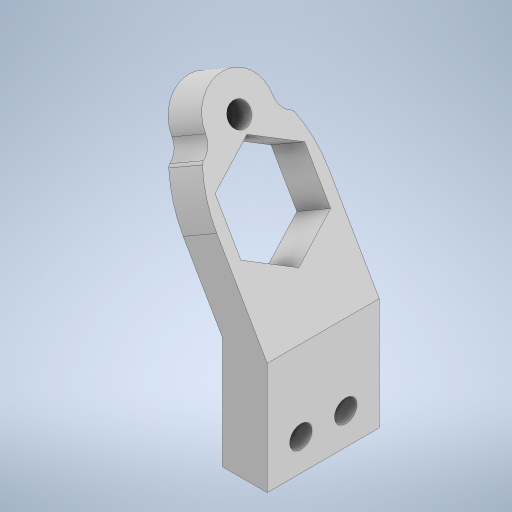
# Autodesk Inventor part: 6 - Part  5
Saved by Autodesk Inventor 2024 (Build 280153000, 153)
## iProperties
Created: 2024-04-21
Part Number: 6 - Part  5
Material: Generic
Document SubType Name: Modeling
Designer: Ricsi
Density: 1 g/cm^3
Appearance: Default
Author: Ricsi
Autodesk Inventor part; units mm, degrees
ref_plane "YZ Plane" through (0, 0, 0) normal (1, 0, 0) x (0, 1, 0)
ref_plane "XZ Plane" through (0, 0, 0) normal (0, 1, 0) x (-1, 0, 0)
ref_plane "XY Plane" through (0, 0, 0) normal (0, 0, 1) x (1, 0, 0)
sketch "Sketch1" plane through (0, 0, 0) normal (1, 0, 0) x (0, 1, 0)
  line L0 (28.0764, 57.8828) -> (-21.9236, 57.8828)
  line L1 (-21.9236, 57.8828) -> (-21.9236, 7.8828)
  line L2 (-21.9236, 7.8828) -> (28.0764, 7.8828)
  line L3 (28.0764, 7.8828) -> (28.0764, 57.8828)
  circle A0 centre (-7.7792, 22.8828) radius 5
  circle A1 centre (-7.7792, 42.8828) radius 5
  point P0 (0, 0)
  dimension "d0" = 50
  dimension "d1" = 50
  dimension "d3" = 10
  dimension "d5" = 10
  constraints: 8 end point, 2 centre point, 2 parallel, 1 horizontal, 1 perpendicular
  measures "d0" distance of L2.end L1.end
  measures "d1" distance of L1.end L0.end
  measures "d3" diameter of A0
  measures "d5" diameter of A1
extrude "Extrusion1" add sketch "Sketch1" along normal blind 20
sketch "Sketch2" plane through (0, -21.9236, 57.8828) normal (0, 0, 1) x (1, 0, 0)
  line L0 (20, 0) -> (20, 50) projected
  line L1 (20, 50) -> (-25, 127.9423)
  line L2 (20, 50) -> (110, 50) construction
  line L3 (0, 50) -> (-45, 127.9423)
  line L4 (0, 50) -> (90, 50) construction
  line L5 (-45, 127.9423) -> (-25, 127.9423)
  line L6 (0, 50) -> (20, 50)
  point P0 (0, 21.9236)
  dimension "d8" = 90
  dimension "d9" = 120
  dimension "d10" = 90
  dimension "d11" = 120
  constraints: 12 end point, 2 equal length, 2 horizontal, 1 collinear
  measures "d8" distance of L0.end L1.end
  measures "d9" angle of L2 L1
  measures "d10" distance of L3.start L3.end
  measures "d11" angle of L4 L3
extrude "Extrusion2" add sketch "Sketch2" against normal blind 50
sketch "Sketch3" plane through (20, 28.0764, 57.8828) normal (0.866, 0.5, 0) x (0, 0, -1)
  line L0 (0, 0) -> (0, -43.3013) projected
  line L1 (0, 0) -> (0, 90) projected
  arc A0 (40, 75) -> (10, 75) centre (25, 75) ccw
  line L2 (0, 0) -> (0, 45)
  line L3 (50, 0) -> (0, 0) projected
  line L4 (0, 0) -> (50, 0)
  line L5 (50, 0) -> (50, 45)
  arc A1 (5.4018, 67.7593) -> (10, 75) centre (2, 75) ccw
  line L6 (10, 75) -> (2, 75) construction
  line L7 (4.7362, 67.4825) -> (2, 75) construction
  arc A2 (40, 75) -> (44.5982, 67.7593) centre (48, 75) ccw
  line L8 (40, 75) -> (48, 75) construction
  line L9 (45.2638, 67.4825) -> (48, 75) construction
  arc A3 (4.4105, 66.7289) -> (0, 45) centre (55.73, 45) ccw
  arc A4 (50, 45) -> (45.5895, 66.7289) centre (-5.73, 45) ccw
  arc A5 (5.4018, 67.7593) -> (4.4105, 66.7289) centre (6.2523, 65.9491) ccw
  arc A6 (45.5895, 66.7289) -> (44.5982, 67.7593) centre (43.7477, 65.9491) ccw
  line L10 (25, 90) -> (0, 90)
  line L11 (0, 90) -> (0, 45)
  line L12 (50, 90) -> (50, 0) projected
  line L13 (50, 90) -> (50, 45)
  line L14 (25, 90) -> (50, 90)
  point P0 (57.8828, -14.3149)
  dimension "d18" = 45
  dimension "d19" = 45
  dimension "d20" = 8
  dimension "d21" = 70
  dimension "d22" = 8
  dimension "d23" = 70
  dimension "d24" = 2
  dimension "d25" = 2
  constraints: 22 end point, 20 point on circle, 9 tangent, 7 centre point, 2 collinear, 2 midpoint, 2 perpendicular
  measures "d18" distance of L0.start L2.end
  measures "d19" distance of L3.start L5.end
  measures "d20" radius of A1
  measures "d21" angle of L7 L6
  measures "d22" radius of A2
  measures "d23" angle of L8 L9
  measures "d24" radius of A5
  measures "d25" radius of A6
extrude "Extrusion3" cut sketch "Sketch3" against normal blind 50 contours L1 L10 A0 A1 A5 A3 | A4 A6 A2 A0 L14 L12
sketch "Sketch4" plane through (-40, 97.3585, 32.8828) normal (0.5, -0.866, 0) x (0.866, 0.5, 0)
  line L0 (17.3205, 25) -> (17.3205, 0) projected
  line L1 (17.3205, 0) -> (17.3205, -25) projected
  line L2 (17.3205, 25) -> (17.3205, -25)
  line L3 (17.3205, -25) -> (-0.3461, -25)
  line L4 (-0.3461, -25) -> (-0.3461, 25)
  line L5 (17.3205, 25) -> (0, 25) projected
  line L6 (-0.3461, 25) -> (17.3205, 25)
  point P0 (-14.0382, -32.8828)
  point P1 (0, 25)
  constraints: 8 end point, 3 perpendicular, 1 collinear
extrude "Extrusion4" cut sketch "Sketch4" against normal blind 50
sketch "Sketch5" plane through (20, 28.0764, 57.8828) normal (0.866, 0.5, 0) x (0, 0, -1)
  line L0 (50, 0) -> (0, 0) projected
  circle A0 centre (25, 75) radius 5
  point P0 (57.8828, -14.3149)
  dimension "d32" = 10
  constraints: 1 centre point
  measures "d32" diameter of A0
extrude "Extrusion5" cut sketch "Sketch5" against normal blind 50
sketch "Sketch6" plane through (20, 28.0764, 57.8828) normal (0.866, 0.5, 0) x (0, 0, -1)
  line L0 (0, 0) -> (0, 45) projected
  line L1 (50, 0) -> (0, 0) projected
  line L2 (25, 68.094) -> (45, 56.547)
  line L3 (45, 56.547) -> (45, 33.453)
  line L4 (45, 33.453) -> (25, 21.906)
  line L5 (25, 21.906) -> (5, 33.453)
  line L6 (5, 33.453) -> (5, 56.547)
  line L7 (5, 56.547) -> (25, 68.094)
  point P0 (57.8828, -14.3149)
  point P1 (25, 45)
  point P2 (45, 45)
  point P3 (5, 45)
  dimension "d37" = 40
  constraints: 12 end point, 2 midpoint, 13 other
  measures "d37" distance of point (45, 45) point (5, 45)
extrude "Extrusion6" cut sketch "Sketch6" against normal blind 30
body "Solid1"
